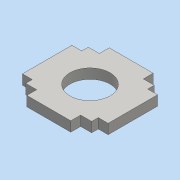
# Autodesk Inventor part: Camera-Holder_Bearing-Ring-Outer
Saved by Autodesk Inventor 2016 SP1 (Build 200210100, 210)
## iProperties
Created: 2016-01-20
Part Number: Camera-Holder_Bearing-Ring-Outer
Material: Generic
Document SubType Name: Modeling
Designer: Mohamed A.
Density: 1 g/cm^3
Appearance: Default
Author: Mohamed A.
Autodesk Inventor part; units mm, degrees
ref_plane "YZ Plane" through (0, 0, 0) normal (1, 0, 0) x (0, 1, 0)
ref_plane "XZ Plane" through (0, 0, 0) normal (0, 1, 0) x (-1, 0, 0)
ref_plane "XY Plane" through (0, 0, 0) normal (0, 0, 1) x (1, 0, 0)
sketch "Sketch1" plane through (0, 0, 0) normal (0, 0, 1) x (1, 0, 0)
  circle A0 centre (0, 0) radius 6.096
  line L0 (13, 7.5) -> (10, 7.5)
  line L1 (10, 7.5) -> (10, 9.5)
  line L2 (10, -9.5) -> (10, -7.5)
  line L3 (10, -7.5) -> (13, -7.5)
  line L4 (-6.6667, -12.5) -> (-6.6667, -9.5)
  line L5 (-6.6667, -9.5) -> (-10, -9.5)
  line L6 (6.6667, -12.5) -> (6.6667, -9.5)
  line L7 (6.6667, -9.5) -> (10, -9.5)
  line L8 (-13, -7.5) -> (-10, -7.5)
  line L9 (-10, -7.5) -> (-10, -9.5)
  line L10 (-13, 7.5) -> (-10, 7.5)
  line L11 (-10, 7.5) -> (-10, 9.5)
  line L12 (-6.6667, 12.5) -> (-6.6667, 9.5)
  line L13 (-6.6667, 9.5) -> (-10, 9.5)
  line L14 (10, 9.5) -> (6.6667, 9.5)
  line L15 (6.6667, 9.5) -> (6.6667, 12.5)
  line L16 (-6.6667, 12.5) -> (6.6667, 12.5)
  line L17 (-13, -7.5) -> (-13, 7.5)
  line L18 (6.6667, -12.5) -> (-6.6667, -12.5)
  line L19 (13, -7.5) -> (13, 7.5)
  line L20 (-20.9424, 0) -> (31.3224, 0) construction
  line L21 (0, 16.7256) -> (0, -15.9648) construction
  dimension "d0" = 12.192
  dimension "d3" = 3
  dimension "d5" = 3
  dimension "d6" = 3
  dimension "d7" = 15
  dimension "d9" = 13.3333
  dimension "d15" = 25
  dimension "d16" = 3
  dimension "d17" = 20
  dimension "d18" = 20
  constraints: 44 end point, 12 point on line, 8 perpendicular, 4 horizontal, 3 collinear, 2 vertical, 1 centre point, 1 coincident, 1 parallel, 3 other
  measures "d0" diameter of A0
  measures "d3" distance of L0.start L0.end
  measures "d5" distance of L8.start L8.end
  measures "d6" distance of L12.start L12.end
  measures "d7" distance between parallel lines of L3 L0
  measures "d9" distance between parallel lines of L12 L15
  measures "d15" distance between parallel lines of L18 L16
  measures "d16" distance of L6.start L6.end
  measures "d17" distance between parallel lines of L11 L1
  measures "d18" distance between parallel lines of L2 L9
extrude "Extrusion1" add sketch "Sketch1" along normal blind 3
equation "\"d9\" = 0.666667 * d17"
body "Solid1"
